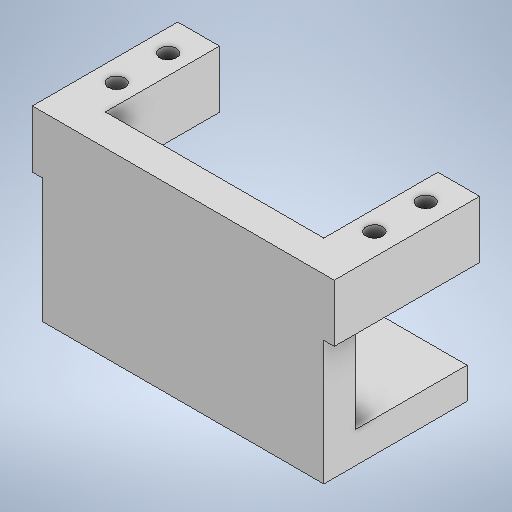
# Autodesk Inventor part: MG996RServoHolder
Saved by Autodesk Inventor 2025.1 (Build 291241020, 241B)
## iProperties
Created: 2021-12-15
Part Number: MG996RServoHolder
Material: 钢
Document SubType Name: Modeling
Designer: omiye
Density: 7.85 g/cm^3
Appearance: Default
Mass: 144.969 g
Surface Area: 93.6221 cm^2
Volume: 18.4674 cm^3
Sending System: Autodesk Translation Framework v10.10.0.1391
Preprocessor: ST-DEVELOPER v18.1
Title: C:/Users/23714/Desktop/Servo Motor MG996R_ 一字摇臂.step
Autodesk Inventor part; units mm, degrees
ref_plane "YZ Plane" through (0, 0, 0) normal (1, 0, 0) x (0, 1, 0)
ref_plane "XZ Plane" through (0, 0, 0) normal (0, 1, 0) x (-1, 0, 0)
ref_plane "XY Plane" through (0, 0, 0) normal (0, 0, 1) x (1, 0, 0)
ref_plane "Work Plane1" through (-19.25, -0.5, 9.85) normal (0, 0, 1) x (1, 0, 0)
sketch "Sketch1" plane through (-19.25, -0.5, 9.85) normal (0, 0, 1) x (1, 0, 0)
  line L0 (-0.695, -27.8) -> (39.2, -27.8)
  line L1 (39.2, -27.8) -> (39.2, 8.9608)
  line L2 (39.2, 8.9608) -> (-0.695, 8.9608)
  line L3 (-0.695, 8.9608) -> (-0.695, -27.8)
  point P0 (19.25, 0.5)
  constraints: 8 end point, 2 parallel, 1 horizontal, 1 perpendicular
extrude "Extrusion1" add sketch "Sketch1" along normal blind 3
ref_plane "Work Plane2" through (-19.25, -0.5, 12.85) normal (0, 0, 1) x (1, 0, 0)
sketch "Sketch2" plane through (-19.25, -0.5, 12.85) normal (0, 0, 1) x (1, 0, 0)
  line L0 (39.2, -27.8) -> (39.2, 8.9608) projected
  line L1 (39.2, -27.8) -> (-0.695, -27.8)
  line L2 (-0.695, -27.8) -> (-0.695, 8.9608)
  line L3 (-0.695, 8.9608) -> (39.2, 8.9608)
  line L4 (39.2, 8.9608) -> (39.2, -27.8)
  point P0 (19.25, 0.5)
  point P1 (39.2, 8.9608)
  constraints: 8 end point, 2 parallel, 1 horizontal, 1 perpendicular
extrude "Extrusion2" add sketch "Sketch2" along normal blind 5
ref_plane "Work Plane4" through (19.95, -28.3, 9.85) normal (1, 0, 0) x (0, 0, -1)
sketch "Sketch3" plane through (19.95, -28.3, 9.85) normal (1, 0, 0) x (0, 0, -1)
  line L0 (0, 0) -> (0, 36.7608) projected
  line L1 (0, 0) -> (-8, 0) projected
  line L2 (0, 36.7608) -> (-2, 36.7608)
  line L3 (-2, 36.7608) -> (-2, 0)
  line L4 (-2, 0) -> (0, 0)
  line L5 (0, 0) -> (0, 36.7608)
  point P0 (9.85, 28.3)
  dimension "d4" = 2
  constraints: 8 end point, 2 parallel, 1 horizontal, 1 perpendicular, 1 point on line
  measures "d4" distance of L4.end L3.end
extrude "Extrusion3" cut sketch "Sketch3" against normal blind 50
ref_plane "Work Plane3" through (19.95, -28.3, 17.85) normal (1, 0, 0) x (0, 0, -1)
sketch "Sketch4" plane through (19.95, -28.3, 17.85) normal (1, 0, 0) x (0, 0, -1)
  line L0 (6, 0) -> (0, 0) projected
  line L1 (6, 36.7608) -> (0, 36.7608) projected
  line L2 (0, 0) -> (1, 0)
  line L3 (1, 0) -> (1, 36.7608)
  line L4 (1, 36.7608) -> (0, 36.7608)
  line L5 (0, 36.7608) -> (0, 0)
  point P0 (17.85, 28.3)
  point P1 (1, 0)
  dimension "d7" = 1
  constraints: 8 end point, 2 parallel, 1 horizontal, 1 perpendicular, 1 point on line
  measures "d7" distance of L4.end L3.end
extrude "Extrusion4" cut sketch "Sketch4" against normal blind 50
ref_plane "Work Plane5" through (19.95, -28.3, 11.85) normal (1, 0, 0) x (0, 0, -1)
sketch "Sketch5" plane through (19.95, -28.3, 11.85) normal (1, 0, 0) x (0, 0, -1)
  line L0 (-5, 36.7608) -> (-5, 0) projected
  line L1 (0, 0) -> (0, 36.7608) projected
  line L2 (-5, 36.7608) -> (0, 36.7608)
  line L3 (0, 36.7608) -> (0, 0)
  line L4 (0, 0) -> (-5, 0)
  line L5 (-5, 0) -> (-5, 36.7608)
  point P0 (11.85, 28.3)
  constraints: 8 end point, 2 parallel, 1 horizontal, 1 perpendicular
extrude "Extrusion5" add sketch "Sketch5" along normal blind 7
ref_plane "Work Plane6" through (-19.945, -28.3, 11.85) normal (0, 0, -1) x (-1, 0, 0)
sketch "Sketch6" plane through (-19.945, -28.3, 11.85) normal (0, 0, -1) x (-1, 0, 0)
  line L0 (-46.895, 0) -> (-46.895, 36.7608) projected
  line L1 (-46.895, 27.8459) -> (-40.895, 27.8459)
  line L2 (-40.895, 27.8459) -> (-40.895, 11.8459)
  line L3 (-40.895, 11.8459) -> (-46.895, 11.8459)
  line L4 (-46.895, 11.8459) -> (-46.895, 27.8459)
  point P0 (-19.945, 28.3)
  dimension "d12" = 6
  dimension "d13" = 16
  constraints: 8 end point, 2 parallel, 1 horizontal, 1 perpendicular, 1 point on line
  measures "d12" distance of L2.end L3.end
  measures "d13" distance of L1.end L2.end
extrude "Extrusion6" add sketch "Sketch6" along normal blind 22.875
sketch "Sketch7" plane through (20.95, -0.4541, 11.85) normal (0, 1, 0) x (1, 0, 0)
  arc A0 (5.4164, 8.2173) -> (5.4164, 5.6327) centre (3.7611, 6.925) ccw projected
  circle A1 centre (3.7611, 6.925) radius 2.5
  arc A2 (5.4164, 18.0673) -> (5.4164, 15.4827) centre (3.7611, 16.775) ccw projected
  circle A3 centre (3.7611, 16.775) radius 2.5
  point P0 (-20.95, 11.85)
  dimension "d16" = 5
  dimension "d17" = 5
  constraints: 2 centre point, 2 coincident
  measures "d16" diameter of A1
  measures "d17" diameter of A3
extrude "Extrusion7" cut sketch "Sketch7" against normal blind 22.875
ref_plane "Work Plane7" through (26.95, -28.3, 11.85) normal (1, 0, 0) x (0, 0, -1)
sketch "Sketch8" plane through (26.95, -28.3, 11.85) normal (1, 0, 0) x (0, 0, -1)
  line L0 (0, 11.8459) -> (22.875, 11.8459) projected
  line L1 (22.875, 27.8459) -> (22.875, 11.8459) projected
  line L2 (0, 11.8459) -> (22.875, 11.8459)
  line L3 (22.875, 11.8459) -> (22.875, 16.8459)
  line L4 (22.875, 16.8459) -> (0, 16.8459)
  line L5 (0, 16.8459) -> (0, 11.8459)
  point P0 (11.85, 28.3)
  dimension "d20" = 5
  constraints: 8 end point, 2 parallel, 1 horizontal, 1 perpendicular, 1 point on line
  measures "d20" distance of L3.end L2.end
extrude "Extrusion8" cut sketch "Sketch8" against normal blind 6.7
ref_plane "Work Plane8" through (-19.945, -28.3, 11.85) normal (-1, 0, 0) x (0, 0, 1)
sketch "Sketch9" plane through (-19.945, -28.3, 11.85) normal (-1, 0, 0) x (0, 0, 1)
  line L0 (0, 36.7608) -> (0, 0) projected
  line L1 (5, 0) -> (0, 0) projected
  line L2 (0, 36.7608) -> (5, 36.7608)
  line L3 (5, 36.7608) -> (5, 0)
  line L4 (5, 0) -> (0, 0)
  line L5 (0, 0) -> (0, 36.7608)
  point P0 (-11.85, 28.3)
  constraints: 8 end point, 2 parallel, 1 horizontal, 1 perpendicular
extrude "Extrusion9" add sketch "Sketch9" along normal blind 7
ref_plane "Work Plane10" through (26.95, -0.4541, 11.85) normal (0, 0, -1) x (-1, 0, 0)
sketch "Sketch11" plane through (26.95, -0.4541, 11.85) normal (0, 0, -1) x (-1, 0, 0)
  line L0 (53.895, -27.8459) -> (53.895, 8.9148) projected
  line L1 (53.895, 0) -> (47.895, 0)
  line L2 (47.895, 0) -> (47.895, -11)
  line L3 (47.895, -11) -> (53.895, -11)
  line L4 (53.895, -11) -> (53.895, 0)
  point P0 (26.95, 0.4541)
  dimension "d25" = 6
  constraints: 8 end point, 2 parallel, 1 horizontal, 1 perpendicular, 1 point on line
  measures "d25" distance of L3.end L2.end
extrude "Extrusion10" add sketch "Sketch11" along normal blind 22.875
sketch "Sketch12" plane through (-26.945, -0.4541, 11.85) normal (0, 1, 0) x (1, 0, 0)
  arc A0 (0.5786, 15.4827) -> (0.5786, 18.0673) centre (2.2339, 16.775) ccw projected
  circle A1 centre (2.2339, 16.775) radius 2.5
  arc A2 (0.5786, 5.6327) -> (0.5786, 8.2173) centre (2.2339, 6.925) ccw projected
  circle A3 centre (2.2339, 6.925) radius 2.5
  point P0 (26.945, 11.85)
  dimension "d28" = 5
  dimension "d29" = 5
  constraints: 2 centre point, 2 coincident
  measures "d28" diameter of A1
  measures "d29" diameter of A3
extrude "Extrusion11" cut sketch "Sketch12" against normal blind 22.875
ref_plane "Work Plane11" through (-26.945, -28.3, 11.85) normal (-1, 0, 0) x (0, 0, 1)
sketch "Sketch13" plane through (-26.945, -28.3, 11.85) normal (-1, 0, 0) x (0, 0, 1)
  line L0 (0, 16.8459) -> (0, 27.8459) projected
  line L1 (5, 36.7608) -> (0, 36.7608) projected
  line L2 (0, 27.8459) -> (5, 27.8459)
  line L3 (5, 27.8459) -> (5, 36.7608)
  line L4 (5, 36.7608) -> (0, 36.7608)
  line L5 (0, 36.7608) -> (0, 27.8459)
  point P0 (-11.85, 28.3)
  constraints: 8 end point, 2 parallel, 1 horizontal, 1 perpendicular
extrude "Extrusion12" cut sketch "Sketch13" against normal blind 67.325
ref_plane "Work Plane9" through (26.95, -28.3, 11.85) normal (0, -1, 0) x (1, 0, 0)
sketch "Sketch14" plane through (26.95, -28.3, 11.85) normal (0, -1, 0) x (1, 0, 0)
  line L0 (0, 5) -> (0, 0) projected
  line L1 (0, 5) -> (-53.895, 5) projected
  line L2 (0, 0) -> (-53.895, 0)
  line L3 (-53.895, 0) -> (-53.895, 5)
  line L4 (-53.895, 5) -> (0, 5)
  line L5 (0, 5) -> (0, 0)
  point P0 (-26.95, -11.85)
  constraints: 8 end point, 2 parallel, 1 horizontal, 1 perpendicular
extrude "Extrusion13" add sketch "Sketch14" along normal blind 5
ref_plane "Work Plane12" through (26.95, -11.4541, 11.85) normal (0, 0, -1) x (-1, 0, 0)
sketch "Sketch15" plane through (26.95, -11.4541, 11.85) normal (0, 0, -1) x (-1, 0, 0)
  line L0 (53.895, -21.8459) -> (0, -21.8459) projected
  line L1 (53.895, 11) -> (53.895, -21.8459) projected
  line L2 (0, -21.8459) -> (53.895, -21.8459)
  line L3 (53.895, -21.8459) -> (53.895, -17.8459)
  line L4 (53.895, -17.8459) -> (0, -17.8459)
  line L5 (0, -17.8459) -> (0, -21.8459)
  point P0 (26.95, 11.4541)
  dimension "d36" = 4
  constraints: 8 end point, 2 parallel, 1 horizontal, 1 perpendicular, 1 point on line
  measures "d36" distance of L3.end L2.end
extrude "Extrusion14" add sketch "Sketch15" along normal blind 22.4625
ref_plane "Work Plane13" through (-26.945, -29.3, 11.85) normal (0, 1, 0) x (1, 0, 0)
sketch "Sketch16" plane through (-26.945, -29.3, 11.85) normal (0, 1, 0) x (1, 0, 0)
  line L0 (53.895, 0) -> (53.895, 22.4625) projected
  line L1 (0, 0) -> (0, 22.4625) projected
  line L2 (53.895, 0) -> (0, 0)
  line L3 (0, 0) -> (0, 1)
  line L4 (0, 1) -> (53.895, 1)
  line L5 (53.895, 1) -> (53.895, 0)
  point P0 (26.945, 11.85)
  point P1 (53.895, 1)
  dimension "d39" = 1
  constraints: 8 end point, 2 parallel, 1 horizontal, 1 perpendicular, 1 point on line
  measures "d39" distance of L2.end L3.end
extrude "Extrusion15" add sketch "Sketch16" along normal blind 30
ref_plane "Work Plane14" through (26.95, -28.3, 11.85) normal (1, 0, 0) x (0, 0, -1)
sketch "Sketch17" plane through (26.95, -28.3, 11.85) normal (1, 0, 0) x (0, 0, -1)
  line L0 (0, 29) -> (1, 29) projected
  line L1 (5.8126, 27.8459) -> (1, 27.8459) projected
  line L2 (0, 29) -> (1, 29)
  line L3 (1, 29) -> (1, 27.8459)
  line L4 (1, 27.8459) -> (0, 27.8459)
  line L5 (0, 27.8459) -> (0, 29)
  point P0 (11.85, 28.3)
  constraints: 8 end point, 2 parallel, 1 horizontal, 1 perpendicular
extrude "Extrusion16" cut sketch "Sketch17" against normal blind 100
sketch "Sketch19" plane through (26.95, -33.3, 11.85) normal (0, -1, 0) x (1, 0, 0)
  circle A0 centre (-16.85, -11.85) radius 5
  circle A1 centre (-16.85, -11.85) radius 1.5
  point P0 (-26.95, -11.85)
  dimension "d47" = 10
  dimension "d50" = 3
  constraints: 2 centre point, 1 coincident
  measures "d47" diameter of A0
  measures "d50" diameter of A1
extrude "Extrusion20" cut sketch "Sketch19" against normal blind 10 contours A1
sketch "Sketch20" plane through (26.95, -33.3, 11.85) normal (0, -1, 0) x (1, 0, 0)
  line L0 (-53.895, -22.4625) -> (0, -22.4625) projected
  line L1 (-53.895, 5) -> (-53.895, -22.4625) projected
  line L2 (0, -22.4625) -> (-53.895, -22.4625)
  line L3 (-53.895, -22.4625) -> (-53.895, 5)
  line L4 (-53.895, 5) -> (0, 5)
  line L5 (0, 5) -> (0, -22.4625)
  point P0 (-26.95, -11.85)
  constraints: 8 end point, 2 parallel, 1 horizontal, 1 perpendicular
extrude "Extrusion21" add sketch "Sketch20" along normal blind 2
sketch "Sketch21" plane through (-26.945, -29.3, -10.6125) normal (0, 1, 0) x (1, 0, 0)
  circle A0 centre (37.045, -10.6125) radius 1.5 projected
  circle A1 centre (37.045, -10.6125) radius 1.5
  point P0 (26.945, -10.6125)
  constraints: 1 centre point, 1 coincident
extrude "Extrusion22" cut sketch "Sketch21" against normal blind 10
sketch "Sketch22" plane through (-26.945, -29.3, -10.6125) normal (0, 1, 0) x (1, 0, 0)
  circle A0 centre (37.045, -10.6125) radius 1.5 projected
  circle A1 centre (37.045, -10.6125) radius 2.5
  point P0 (26.945, -10.6125)
  dimension "d59" = 5
  constraints: 1 centre point, 1 coincident
  measures "d59" diameter of A1
extrude "Extrusion23" cut sketch "Sketch22" against normal blind 2
sketch "Sketch23" plane through (-19.945, -28.3, -11.025) normal (0, 0, -1) x (-1, 0, 0)
  line L0 (-46.895, 27.8459) -> (-46.895, 16.8459) projected
  line L1 (-46.895, 27.8459) -> (-48.895, 27.8459)
  line L2 (-48.895, 27.8459) -> (-48.895, 16.8459)
  line L3 (-48.895, 16.8459) -> (-46.895, 16.8459)
  line L4 (-46.895, 16.8459) -> (-46.895, 27.8459)
  line L5 (7, 16.8459) -> (7, 27.8459) projected
  line L6 (7, 27.8459) -> (9, 27.8459)
  line L7 (9, 27.8459) -> (9, 16.8459)
  line L8 (9, 16.8459) -> (7, 16.8459)
  line L9 (7, 16.8459) -> (7, 27.8459)
  point P0 (-19.945, 28.3)
  dimension "d62" = 2
  dimension "d63" = 2
  constraints: 16 end point, 4 parallel, 2 horizontal, 2 perpendicular, 1 point on line
  measures "d62" distance of L3.end L2.end
  measures "d63" distance of L7.end L8.end
extrude "Extrusion24" add sketch "Sketch23" against normal up to surface (27.875 mm away)
sketch "Sketch24" plane through (-20.945, -0.4541, 10.85) normal (0, 1, 0) x (1, 0, 0)
  arc A0 (47.895, 7.0374) -> (47.895, 4.8126) centre (45.6561, 5.925) ccw projected
  circle A1 centre (45.6561, 5.925) radius 1.6
  arc A2 (47.895, 16.8874) -> (47.895, 14.6626) centre (45.6561, 15.775) ccw projected
  circle A3 centre (45.6561, 15.775) radius 1.6
  circle A4 centre (45.6561, 5.925) radius 2.5
  circle A5 centre (45.6561, 15.775) radius 2.5
  point P0 (20.945, 10.85)
  point P1 (47.895, 4.8126)
  dimension "d66" = 3.2
  dimension "d67" = 3.2
  constraints: 4 centre point, 4 coincident
  measures "d66" diameter of A1
  measures "d67" diameter of A3
extrude "Extrusion25" add sketch "Sketch24" against normal up to surface (11 mm away)
sketch "Sketch25" plane through (-20.945, -0.4541, 10.85) normal (0, 1, 0) x (1, 0, 0)
  arc A0 (-6, 4.8025) -> (-6, 7.0475) centre (-3.7661, 5.925) ccw projected
  circle A1 centre (-3.7661, 5.925) radius 1.6
  arc A2 (-6, 14.6525) -> (-6, 16.8975) centre (-3.7661, 15.775) ccw projected
  circle A3 centre (-3.7661, 15.775) radius 1.6
  circle A4 centre (-3.7661, 15.775) radius 2.5
  circle A5 centre (-3.7661, 5.925) radius 2.5
  point P0 (20.945, 10.85)
  point P1 (-6, 7.0475)
  dimension "d70" = 3.2
  dimension "d71" = 3.2
  dimension "d72" = 5
  dimension "d73" = 5
  constraints: 4 centre point, 4 coincident
  measures "d70" diameter of A1
  measures "d71" diameter of A3
  measures "d72" diameter of A4
  measures "d73" diameter of A5
extrude "Extrusion26" add sketch "Sketch25" against normal up to surface (11 mm away)
sketch "Sketch26" plane through (26.95, -35.3, 11.85) normal (0, -1, 0) x (1, 0, 0)
  line L0 (-55.895, -22.875) -> (-55.895, 5) projected
  line L1 (-55.895, -11.85) -> (-37.045, -11.85)
  line L2 (-55.895, -11.85) -> (-37.045, -11.85) construction
  circle A0 centre (-37.045, -11.85) radius 1.5
  point P0 (-26.95, -11.85)
  dimension "d76" = 18.85
  dimension "d77" = 0
  dimension "d78" = 3
  constraints: 4 end point, 1 centre point, 1 coincident, 1 collinear, 1 horizontal, 1 perpendicular, 1 point on line
  measures "d76" distance of L1.start L1.end
  measures "d77" distance between parallel lines of L1 L2
  measures "d78" diameter of A0
extrude "Extrusion27" cut sketch "Sketch26" against normal blind 10
sketch "Sketch27" plane through (-26.945, -29.3, -10.6125) normal (0, 1, 0) x (1, 0, 0)
  circle A0 centre (16.85, -10.6125) radius 1.5 projected
  circle A1 centre (16.85, -10.6125) radius 2.5
  point P0 (26.945, -10.6125)
  dimension "d81" = 5
  constraints: 1 centre point, 1 coincident
  measures "d81" diameter of A1
extrude "Extrusion28" cut sketch "Sketch27" against normal up to surface (2 mm away)
body "Solid1"
body "Solid13"
